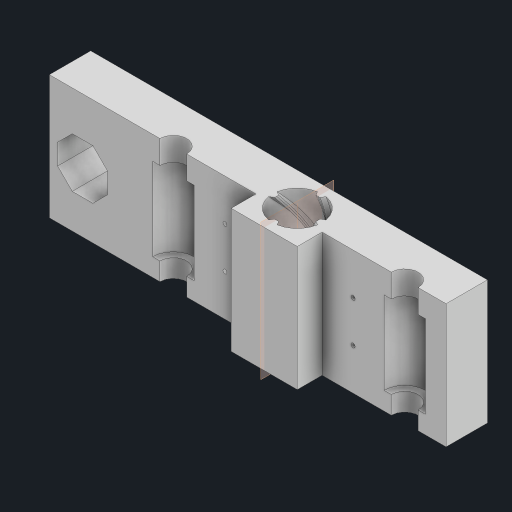
# Autodesk Inventor part: carriage_slider_bottom
Saved by Autodesk Inventor 2024 (Build 280153000, 153)
## iProperties
Created: 2024-06-23
Part Number: carriage_slider_bottom
Material: Generic
Document SubType Name: Modeling
Designer: mihir
Density: 1 g/cm^3
Appearance: Default
Author: mihir
Autodesk Inventor part; units mm, degrees
ref_plane "YZ Plane" through (0, 0, 0) normal (1, 0, 0) x (0, 1, 0)
ref_plane "XZ Plane" through (0, 0, 0) normal (0, 1, 0) x (-1, 0, 0)
ref_plane "XY Plane" through (0, 0, 0) normal (0, 0, 1) x (1, 0, 0)
sketch "Sketch1" plane through (0, 0, 0) normal (0, 1, 0) x (-1, 0, 0)
  line L0 (-8, 8) -> (8, 8)
  line L1 (8, 8) -> (8, -8)
  line L2 (8, -8) -> (-8, -8)
  line L3 (-8, -8) -> (-8, 8)
  line L4 (-8, 8) -> (8, -8) construction
  line L5 (8, 8) -> (-8, -8) construction
  circle A0 centre (0, 0) radius 6
  dimension "d0" = 12
  dimension "d1" = 8
  constraints: 12 end point, 2 midpoint, 2 parallel, 2 perpendicular, 1 centre point, 1 coincident, 1 horizontal
  measures "d0" diameter of A0
  measures "d1" distance from line of L1 A0.centre
extrude "Extrusion1" add sketch "Sketch1" along normal blind 30
sketch "Sketch2" plane through (0, 30, 0) normal (0, 1, 0) x (1, 0, 0)
  circle A0 centre (0, 0) radius 5 construction
  circle A1 centre (0, 0) radius 6 projected
  line L0 (0, -6) -> (-1.0774, -6)
  line L1 (-1.0774, -6) -> (-0.5, -5)
  line L2 (-0.5, -5) -> (0, -5)
  line L3 (0, -6) -> (0, -5)
  line L4 (0, -5) -> (0, 0) construction
  line L5 (0, -6) -> (1.0774, -6)
  line L6 (1.0774, -6) -> (0.5, -5)
  line L7 (0.5, -5) -> (0, -5)
  dimension "d4" = 10
  dimension "d5" = 120
  dimension "d6" = 0.5
  constraints: 16 end point, 2 horizontal, 2 symmetric about line, 2 vertical, 2 vertical alignment, 1 coincident, 3 other
  measures "d6" distance of L1.end L2.end
coil "Coil1" sketch "Sketch2" operation add axis through (0, 30, 0) along (0, -1, 0) pitch 40 turns 0.75 hand right contours L1 L2 L3 A1 | A1 L0 L1 | L6 L5 A1 | A1 L3 L7 L6
pattern_circular "Circular Pattern1" count 4 over 360 about axis through (0, 30, 0) along (0, -1, 0) of "Coil1"
sketch "Sketch3" plane through (8, 0, -8) normal (0, 0, -1) x (-1, 0, 0)
  line L0 (16, 0) -> (16, 30) projected
  line L1 (16, 30) -> (66, 30)
  line L2 (66, 30) -> (66, 0)
  line L3 (66, 0) -> (16, 0)
  line L4 (16, 0) -> (16, 30)
  line L5 (0, 0) -> (0, 30) projected
  line L6 (0, 30) -> (-30, 30)
  line L7 (-30, 30) -> (-30, 0)
  line L8 (-30, 0) -> (0, 0)
  line L9 (0, 0) -> (0, 30)
  line L10 (16, 0) -> (0, 0) projected
  point P0 (8, 0)
  point P1 (0, 0)
  point P2 (16, 0)
  dimension "d18" = 50
  dimension "d19" = 30
  constraints: 16 end point, 4 parallel, 2 collinear, 2 horizontal, 2 perpendicular
  measures "d18" distance of L2.end L3.end
  measures "d19" distance of L7.end L8.end
extrude "Extrusion2" add sketch "Sketch3" against normal blind 10
sketch "Sketch5" plane through (8, 0, 2) normal (0, 0, 1) x (1, 0, 0)
  line L0 (15, 4.357) -> (20, 4.357)
  line L1 (20, 4.357) -> (20, 24.357)
  line L2 (20, 24.357) -> (15, 24.357)
  line L3 (15, 24.357) -> (15, 4.357)
  line L4 (30, 0) -> (30, 30) projected
  point P0 (-8, 0)
  dimension "d22" = 20
  dimension "d23" = 5
  dimension "d24" = 15
  constraints: 8 end point, 2 parallel, 1 horizontal, 1 perpendicular
  measures "d22" distance of L2.end L0.start
  measures "d23" distance of L1.end L2.end
  measures "d24" distance from line of L4 L0.start
revolve "Revolution1" cut sketch "Sketch5" angle 360 about axis through (28, 4.357, 2) along (0, 1, 0)
sketch "Sketch6" plane through (8, 0, 2) normal (0, 0, 1) x (1, 0, 0)
  line L0 (7.5, 10) -> (7.5, 20) construction
  line L1 (0, 0) -> (0, 30) construction
  line L2 (0, 15) -> (15, 15) construction
  line L3 (15, 4.357) -> (15, 24.357) construction
  point P0 (-8, 0)
  point P1 (7.5, 15)
  dimension "d26" = 10
  constraints: 4 end point, 3 midpoint, 1 horizontal, 1 point on line, 1 vertical
  measures "d26" distance of L0.end L0.start
hole "Hole1" at (15.5, 10, 2) at (15.5, 20, 2) direction (0, 0, -1) diameter 1 depth 10 tip angle 118
ref_plane "Work Plane1" through (0, 0, 8) normal (1, 0, 0) x (0, 0, -1)
mirror "Mirror1" about plane through (0, 0, 8) normal (1, 0, 0) of "Revolution1", "Hole1"
sketch "Sketch7" plane through (8, 0, 2) normal (0, 0, 1) x (1, 0, 0)
  line L0 (-60.4645, 20.3925) -> (-55.4645, 20.3925)
  line L1 (-55.4645, 20.3925) -> (-51.9289, 16.857)
  line L2 (-51.9289, 16.857) -> (-51.9289, 11.857)
  line L3 (-51.9289, 11.857) -> (-55.4645, 8.3214)
  line L4 (-55.4645, 8.3214) -> (-60.4645, 8.3214)
  line L5 (-60.4645, 8.3214) -> (-64, 11.857)
  line L6 (-64, 11.857) -> (-64, 16.857)
  line L7 (-64, 16.857) -> (-60.4645, 20.3925)
  line L8 (-41, 4.357) -> (-41, 24.357) construction
  line L9 (-41, 14.357) -> (-66, 14.357) construction
  line L10 (-66, 30) -> (-66, 0) construction
  point P0 (-8, 0)
  point P1 (-57.9645, 14.357)
  dimension "d34" = 2
  dimension "d35" = 5
  constraints: 18 end point, 2 point on line, 1 horizontal, 1 midpoint, 1 perpendicular, 17 other
  measures "d34" distance between parallel lines of L10 L6
  measures "d35" distance of L5.end L6.end
extrude "Extrusion3" cut sketch "Sketch7" against normal up to surface (10 mm away)
sketch "Sketch8" plane through (38, 0, -8) normal (0, 0, -1) x (-1, 0, 0)
  line L0 (94, 16.857) -> (94, 11.857) projected
  line L1 (90.4645, 20.3925) -> (94, 16.857) projected
  line L2 (85.4645, 20.3925) -> (90.4645, 20.3925) projected
  line L3 (81.9289, 16.857) -> (85.4645, 20.3925) projected
  line L4 (81.9289, 11.857) -> (81.9289, 16.857) projected
  line L5 (85.4645, 8.3214) -> (81.9289, 11.857) projected
  line L6 (90.4645, 8.3214) -> (85.4645, 8.3214) projected
  line L7 (94, 11.857) -> (90.4645, 8.3214) projected
  line L8 (94, 11.857) -> (94, 16.857)
  line L9 (90.4645, 20.3925) -> (85.4645, 20.3925)
  line L10 (90.4645, 20.3925) -> (94, 16.857)
  line L11 (85.4645, 20.3925) -> (81.9289, 16.857)
  line L12 (81.9289, 16.857) -> (81.9289, 11.857)
  line L13 (81.9289, 11.857) -> (85.4645, 8.3214)
  line L14 (90.4645, 8.3214) -> (94, 11.857)
  line L15 (90.4645, 8.3214) -> (85.4645, 8.3214)
  circle A0 centre (87.9645, 14.357) radius 4
  circle A1 centre (87.9645, 14.357) radius 6.0355 construction
  point P0 (38, 0)
  dimension "d38" = 8
  constraints: 16 end point, 6 collinear, 3 tangent, 2 centre point, 1 concentric, 1 perpendicular
  measures "d38" diameter of A0
extrude "Extrusion4" add sketch "Sketch8" against normal blind 1
sketch "Sketch9" plane through (0, 0, 0) normal (0, -1, 0) x (1, 0, 0)
  arc A0 (23, 2) -> (33, 2) centre (28, 2) ccw projected
  line L0 (8, 2) -> (38, 2) projected
  arc A1 (24.75, 2) -> (31.25, 2) centre (28, 2) ccw
  line L1 (31.25, 2) -> (24.75, 2)
  point P0 (0, 0)
  point P1 (31.25, 2)
  dimension "d41" = 3.25
  constraints: 2 end point, 2 point on circle, 1 centre point, 1 coincident, 1 collinear, 1 point on line
  measures "d41" radius of A1
extrude "Extrusion5" cut sketch "Sketch9" against normal up to surface (30 mm away) contours L0 A1
mirror "Mirror2" about plane through (0, 0, 8) normal (1, 0, 0) of "Extrusion5"
equation "\"d0\" = lead_screw_outer_diameter"
equation "\"d2\" = slider_width"
equation "\"d4\" = lead_screw_diameter"
equation "\"d5\" = screw_profile_angle"
equation "\"d6\" = 0.5 * screw_profile_width"
equation "\"d7\" = screw_pitch"
equation "\"d18\" = slider_length_needle"
equation "\"d19\" = slider_length_back"
equation "\"d20\" = slider_thickness"
equation "\"d22\" = bearing_length"
equation "\"d23\" = 0.5 * bearing_diameter"
equation "\"d24\" = bearing_dist"
equation "\"d26\" = screw_dist"
equation "\"d27\" = screw_diameter"
equation "\"d34\" = octagon_dist"
equation "\"d35\" = octagon_length"
equation "\"d36\" = slider_thickness"
equation "\"d38\" = needle_hole_diameter"
equation "\"d41\" = 0.5 * rod_free_tolerance + 0.5 * rod_diameter"
equation "\"lead_screw_outer_diameter\" = 12"
equation "\"screw_profile_width\" = 1"
equation "\"screw_profile_angle\" = 120deg"
equation "\"screw_pitch\" = 40"
equation "\"slider_width\" = 30"
equation "\"slider_length_needle\" = 50"
equation "\"slider_thickness\" = 10"
equation "\"bearing_length\" = 20"
equation "\"screw_diameter\" = 1"
equation "\"bearing_dist\" = 15"
equation "\"slider_length_back\" = 30"
equation "\"screw_dist\" = 10"
equation "\"octagon_length\" = 5"
equation "\"octagon_dist\" = 2"
equation "\"needle_hole_diameter\" = 8"
equation "\"rod_diameter\" = 6"
equation "\"rod_free_tolerance\" = 0.5"
equation "\"lead_screw_diameter\" = 10"
equation "\"bearing_diameter\" = 10"
body "Solid1"
